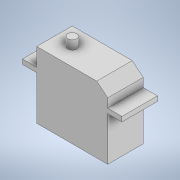
# Autodesk Inventor part: servospt35
Saved by Autodesk Inventor 2020 (Build 240168000, 168)
## iProperties
Created: 2021-03-17
Part Number: servospt35
Material: Generic
Document SubType Name: Modeling
Designer: super
Density: 1 g/cm^3
Appearance: Default
Author: super
Autodesk Inventor part; units mm, degrees
ref_plane "YZ Plane" through (0, 0, 0) normal (1, 0, 0) x (0, 1, 0)
ref_plane "XZ Plane" through (0, 0, 0) normal (0, 1, 0) x (-1, 0, 0)
ref_plane "XY Plane" through (0, 0, 0) normal (0, 0, 1) x (1, 0, 0)
sketch "Sketch1" plane through (0, 0, 0) normal (0, 0, 1) x (1, 0, 0)
  line L0 (0, 0) -> (40, 0)
  line L1 (40, 0) -> (40, 24.7)
  line L2 (0, 24.7) -> (0, 0)
  line L3 (0, 24.7) -> (-8, 24.7)
  line L4 (-8, 24.7) -> (-8, 27.4)
  line L5 (-8, 27.4) -> (0, 27.4)
  line L6 (0, 27.4) -> (0, 37.5)
  line L7 (40, 27.4) -> (48, 27.4)
  line L8 (48, 27.4) -> (48, 24.7)
  line L9 (48, 24.7) -> (40, 24.7)
  line L10 (40, 27.4) -> (40, 32.4)
  line L11 (0, 37.5) -> (33.7964, 37.5)
  line L12 (33.7964, 37.5) -> (40, 32.4)
  dimension "d0" = 40
  dimension "d1" = 24.7
  dimension "d2" = 2.7
  dimension "d9" = 37.5
  dimension "d13" = 8
  dimension "d14" = 8
  dimension "d15" = 8
  dimension "d16" = 5
  constraints: 26 end point, 4 horizontal, 2 perpendicular, 2 point on line, 2 vertical, 1 parallel
  measures "d0" distance of L2.start L1.end
  measures "d1" distance of L1.end L0.end
  measures "d2" distance of L3.end L4.end
  measures "d9" distance of L0.start L6.end
  measures "d13" distance of L2.start L3.end
  measures "d14" distance of L7.start L7.end
  measures "d15" distance of L8.end L1.end
  measures "d16" distance of L7.start L10.end
extrude "Extrusion1" add sketch "Sketch1" against normal blind 20
sketch "Sketch3" plane through (0, 37.5, 0) normal (0, 1, 0) x (1, 0, 0)
  circle A0 centre (10, 10) radius 2.5
  line L0 (0, 0) -> (0, 20) projected
  line L1 (0, 20) -> (33.7964, 20) projected
  dimension "d17" = 5
  dimension "d18" = 10
  dimension "d19" = 10
  constraints: 1 centre point
  measures "d17" diameter of A0
  measures "d18" distance from line of L0 A0.centre
  measures "d19" distance from line of L1 A0.centre
extrude "Extrusion3" add sketch "Sketch3" along normal blind 5
body "Solid1"
